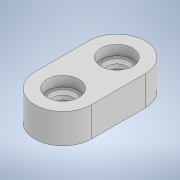
# Autodesk Inventor part: Reduccion_Theta
Saved by Autodesk Inventor 2021 (Build 250183000, 183)
## iProperties
Created: 2021-01-12
Part Number: Reduccion_Theta
Material: Generic
Document SubType Name: Modeling
Designer: jorge
Density: 1 g/cm^3
Appearance: Default
Author: jorge
Autodesk Inventor part; units mm, degrees
ref_plane "YZ Plane" through (0, 0, 0) normal (1, 0, 0) x (0, 1, 0)
ref_plane "XZ Plane" through (0, 0, 0) normal (0, 1, 0) x (-1, 0, 0)
ref_plane "XY Plane" through (0, 0, 0) normal (0, 0, 1) x (1, 0, 0)
sketch "Sketch1" plane through (0, 0, 0) normal (0, 1, 0) x (-1, 0, 0)
  circle A0 centre (0, 0) radius 11.2
  circle A1 centre (0, -38) radius 11.2
  circle A2 centre (0, 0) radius 20
  circle A3 centre (0, -38) radius 20
  line L0 (20, 0) -> (20, -38)
  line L1 (-20, 0) -> (-20, -38)
  dimension "d0" = 22.4
  dimension "d1" = 22.4
  dimension "d2" = 0
  dimension "d3" = 38
  dimension "d4" = 40
  dimension "d5" = 40
  constraints: 4 centre point, 4 end point, 4 point on circle, 3 coincident, 2 tangent
  measures "d0" diameter of A0
  measures "d1" diameter of A1
  measures "d2" horizontal distance of point (0, 0) A1.centre
  measures "d3" distance of point (0, 0) A1.centre
  measures "d4" diameter of A2
  measures "d5" diameter of A3
extrude "Extrusion1" add sketch "Sketch1" along normal blind 21
ref_plane "Work Plane1" through (0, 14, 0) normal (0, 1, 0) x (1, 0, 0)
sketch "Sketch2" plane through (0, 14, 0) normal (0, 1, 0) x (1, 0, 0)
  circle A0 centre (0, 0) radius 7
  circle A1 centre (0, 38) radius 11.2 projected
  circle A2 centre (0, 38) radius 7
  circle A3 centre (0, 0) radius 11.1
  dimension "d9" = 14
  dimension "d10" = 14
  constraints: 3 centre point, 3 coincident
  measures "d9" diameter of A0
  measures "d10" diameter of A2
extrude "Extrusion2" add sketch "Sketch2" against normal blind 7
chamfer "Chamfer1" distance 2 angle 45 4 edges at (-7, 14, 0) (-7, 14, -38) (-7, 7, -38) (-7, 7, 0)
body "Solid1"
